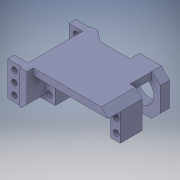
# Autodesk Inventor part: 000.502 - Стяжка
Saved by Autodesk Inventor 2019 (Build 230136000, 136)
## iProperties
Created: 2020-02-29
Part Number: 000.502 - Стяжка
Material: Пластик АБС
Document SubType Name: Modeling
Designer: Петров Иван
Density: 1.06 g/cm^3
Appearance: Грифельно-синий
Author: Петров Иван
Autodesk Inventor part; units mm, degrees
ref_plane "YZ Plane" through (0, 0, 0) normal (1, 0, 0) x (0, 1, 0)
ref_plane "XZ Plane" through (0, 0, 0) normal (0, 1, 0) x (-1, 0, 0)
ref_plane "XY Plane" through (0, 0, 0) normal (0, 0, 1) x (1, 0, 0)
sketch "Эскиз1" plane through (0, 0, 0) normal (0, 1, 0) x (-1, 0, 0)
  line L0 (-20.35, 18.35) -> (-20.35, 12.05)
  line L1 (-20.35, 12.05) -> (-26.35, 12.05)
  line L2 (-26.35, 9.45) -> (-26.35, 12.05)
  line L3 (-20.35, 9.45) -> (-26.35, 9.45)
  line L4 (-20.35, 9.45) -> (-20.35, -16.35)
  line L5 (-20.35, -16.35) -> (20.35, -16.35)
  line L6 (20.35, -16.35) -> (20.35, 9.45)
  line L7 (20.35, 9.45) -> (26.35, 9.45)
  line L8 (26.35, 9.45) -> (26.35, 12.05)
  line L9 (20.35, 12.05) -> (26.35, 12.05)
  line L10 (20.35, 12.05) -> (20.35, 18.35)
  line L11 (20.35, 18.35) -> (-10.35, 18.35)
  line L12 (-10.35, 18.35) -> (-20.35, 18.35)
  line L13 (26.35, 12.05) -> (27.35, 12.05)
  line L14 (26.35, 9.45) -> (26.35, 12.05)
  line L15 (26.35, 9.45) -> (27.35, 9.45)
  line L16 (27.35, 9.45) -> (27.35, 12.05)
  line L17 (-26.35, 12.05) -> (-27.35, 12.05)
  line L18 (-27.35, 9.45) -> (-27.35, 12.05)
  line L19 (-26.35, 9.45) -> (-27.35, 9.45)
  line L20 (-26.35, 9.45) -> (-26.35, 12.05)
  line L21 (-19.55, -17.15) -> (-18.4831, -17.15)
  line L22 (-18.4831, -17.15) -> (-17.3169, -17.15)
  line L23 (-17.3169, -17.15) -> (-15.85, -17.15)
  line L24 (-15.85, -17.15) -> (-15.85, -18.35)
  line L25 (15.85, -18.35) -> (-15.85, -18.35)
  line L26 (15.85, -17.15) -> (15.85, -18.35)
  line L27 (15.85, -17.15) -> (17.3169, -17.15)
  line L28 (17.3169, -17.15) -> (18.4831, -17.15)
  line L29 (18.4831, -17.15) -> (19.55, -17.15)
  line L30 (19.55, -17.15) -> (20.35, -16.35)
  line L31 (-20.35, -16.35) -> (20.35, -16.35)
  line L32 (-19.55, -17.15) -> (-20.35, -16.35)
  line L33 (15.85, -18.35) -> (18.35, -18.35)
  line L34 (-15.85, -18.35) -> (-18.35, -18.35)
  line L35 (18.35, -17.15) -> (18.35, -18.35)
  line L36 (18.35, -18.35) -> (19.55, -17.15)
  line L37 (-19.55, -17.15) -> (-19.65, -17.15)
  line L38 (-18.35, -18.35) -> (-19.55, -17.15)
  line L39 (-7.95, 26.65) -> (-12.75, 26.65)
  line L40 (-10.35, 18.35) -> (-20.35, 18.35)
  line L41 (-10.35, 26.65) -> (-10.35, 18.35)
  line L42 (-27.35, 9.45) -> (27.35, 9.45)
  line L43 (27.35, 9.45) -> (27.35, -19.4732)
  line L44 (27.35, -19.4732) -> (-27.35, -19.4732)
  line L45 (-27.35, -19.4732) -> (-27.35, 9.45)
  line L46 (20.35, 9.45) -> (-20.35, 9.45)
  line L47 (-20.35, 9.45) -> (-20.35, -18.35)
  line L48 (-20.35, -18.35) -> (20.35, -18.35)
  line L49 (20.35, -18.35) -> (20.35, 9.45)
  line L50 (-20.35, -16.35) -> (-27.35, -16.35)
  line L51 (-27.35, -16.35) -> (-27.35, -6.7017)
  line L52 (-27.35, -6.7017) -> (-20.35, -6.7017)
  line L53 (-20.35, -6.7017) -> (-20.35, -16.35)
  line L54 (27.35, -16.35) -> (27.35, -6.7017)
  line L55 (27.35, -6.7017) -> (20.35, -6.7017)
  line L56 (20.35, -6.7017) -> (20.35, -16.35)
  line L57 (27.35, 9.45) -> (20.35, 9.45)
  line L58 (20.35, 9.45) -> (20.35, -6.7017)
  line L59 (20.35, -6.7017) -> (27.35, -6.7017)
  line L60 (27.35, -6.7017) -> (27.35, 9.45)
  line L61 (-20.35, 9.45) -> (-27.35, 9.45)
  line L62 (-27.35, 9.45) -> (-27.35, -6.7017)
  line L63 (-27.35, -6.7017) -> (-20.35, -6.7017)
  line L64 (-20.35, -6.7017) -> (-20.35, 9.45)
  line L65 (27.35, -6.7017) -> (20.35, -6.7017)
  point P0 (0, 0)
  point P1 (0, 0)
  dimension "d0" = 0
  constraints: 132 end point, 12 equal length, 6 perpendicular, 5 horizontal, 4 point on line, 1 midpoint
  measures "d0" distance between parallel lines of L7 L42
extrude "Выдавливание1" add sketch "Эскиз1" along normal blind 20 contours L3 L4 L52 L45 L19 | L7 L15 L43 L55 L6
sketch "Эскиз2" plane through (0, 20, 0) normal (0, 1, 0) x (1, 0, 0)
  line L0 (-27.35, -9.45) -> (-20.35, -9.45) projected
  line L1 (27.35, -9.45) -> (27.35, 6.7017) projected
  line L2 (-27.35, -9.45) -> (27.35, -9.45)
  line L3 (27.35, -9.45) -> (27.35, 6.7017)
  line L4 (27.35, 6.7017) -> (-27.35, 6.7017)
  line L5 (-27.35, 6.7017) -> (-27.35, -9.45)
  point P0 (0, 0)
  constraints: 8 end point, 2 parallel, 1 horizontal, 1 perpendicular
extrude "Выдавливание2" add sketch "Эскиз2" along normal blind 5
sketch "Эскиз3" plane through (20.35, 0, 9.45) normal (0, 0, 1) x (1, 0, 0)
  line L0 (-47.7, 13.75) -> (-47.7, 10.5)
  line L1 (-47.7, 10.5) -> (-40.7, 10.5)
  line L2 (-40.7, 10.5) -> (-40.7, 20)
  line L3 (-40.7, 20) -> (-46.7, 20)
  arc A0 (-46.7, 20) -> (-47.7, 19) centre (-46.7, 19) ccw
  line L4 (-47.7, 19) -> (-47.7, 16.15)
  line L5 (-47.7, 16.15) -> (-46.634, 16.15)
  arc A1 (-46.634, 13.75) -> (-46.634, 16.15) centre (-44.85, 14.95) ccw
  line L6 (-46.634, 13.75) -> (-47.7, 13.75)
  line L7 (-47.7, 9.5) -> (-40.7, 9.5)
  line L8 (-47.7, 9.5) -> (-47.7, 6.25)
  line L9 (-47.7, 6.25) -> (-46.634, 6.25)
  arc A2 (-46.634, 3.85) -> (-46.634, 6.25) centre (-44.85, 5.05) ccw
  line L10 (-46.634, 3.85) -> (-47.7, 3.85)
  line L11 (-47.7, 3.85) -> (-47.7, 1)
  arc A3 (-47.7, 1) -> (-46.7, 0) centre (-46.7, 1) ccw
  line L12 (-46.7, 0) -> (-40.7, 0)
  line L13 (-40.7, 0) -> (-40.7, 9.5)
  line L14 (0, 9.5) -> (7, 9.5)
  line L15 (0, 0) -> (0, 9.5)
  line L16 (6, 0) -> (0, 0)
  arc A4 (6, 0) -> (7, 1) centre (6, 1) ccw
  line L17 (7, 3.85) -> (7, 1)
  line L18 (5.934, 3.85) -> (7, 3.85)
  arc A5 (5.934, 6.25) -> (5.934, 3.85) centre (4.15, 5.05) ccw
  line L19 (7, 6.25) -> (5.934, 6.25)
  line L20 (7, 9.5) -> (7, 6.25)
  line L21 (0, 10.5) -> (0, 20)
  line L22 (0, 10.5) -> (7, 10.5)
  line L23 (7, 13.75) -> (7, 10.5)
  line L24 (5.934, 13.75) -> (7, 13.75)
  arc A6 (5.934, 16.15) -> (5.934, 13.75) centre (4.15, 14.95) ccw
  line L25 (7, 16.15) -> (5.934, 16.15)
  line L26 (7, 19) -> (7, 16.15)
  arc A7 (7, 19) -> (6, 20) centre (6, 19) ccw
  line L27 (0, 20) -> (6, 20)
  line L28 (-40.7, 20) -> (-10, 20)
  line L29 (-10, 20) -> (0, 20)
  line L30 (-10, 0) -> (0, 0)
  line L31 (-40.7, 0) -> (-10, 0)
  circle A8 centre (-10, 10) radius 6.5
  circle A9 centre (-10, 10) radius 5.4
  circle A10 centre (-10, 10) radius 3.4957
  circle A11 centre (-10, 10) radius 3.4957
  circle A12 centre (-44.85, 14.95) radius 2.15
  circle A13 centre (-44.85, 5.05) radius 2.15
  arc A14 (5.934, 16.15) -> (5.934, 13.75) centre (4.15, 14.95) ccw
  circle A15 centre (4.15, 14.95) radius 2.15
  circle A16 centre (4.15, 5.05) radius 2.15
  line L32 (-47.7, 13.75) -> (-47.7, 10.5)
  line L33 (-47.7, 16.15) -> (-47.7, 13.75)
  line L34 (-47.7, 13.75) -> (-47.7, 6.25)
  line L35 (-47.7, 6.25) -> (-47.7, 3.85)
  line L36 (7, 16.15) -> (7, 13.75)
  line L37 (7, 6.25) -> (5.934, 6.25)
  line L38 (7, 6.25) -> (7, 3.85)
  line L39 (0, 20) -> (-40.7, 20) projected
  line L40 (-10, 20) -> (0, 20)
  point P0 (-20.35, 0)
  point P1 (-20.35, 0)
  constraints: 80 end point, 18 point on circle, 15 centre point, 4 coincident, 2 collinear, 2 concentric, 2 vertical, 1 perpendicular, 1 point on line, 6 other
extrude "Выдавливание3" cut sketch "Эскиз3" against normal through all contours A12 A1 | A2 A13 | A16 A5 | A6 A15
sketch "Эскиз4" plane through (0, 25, 0) normal (0, 1, 0) x (1, 0, 0)
  line L0 (20.35, -18.35) -> (20.35, -12.05)
  line L1 (20.35, -12.05) -> (26.35, -12.05)
  line L2 (26.35, -9.45) -> (26.35, -12.05)
  line L3 (20.35, -9.45) -> (26.35, -9.45)
  line L4 (20.35, -9.45) -> (20.35, 16.35)
  line L5 (-20.35, 16.35) -> (-20.35, -9.45)
  line L6 (-20.35, -9.45) -> (-26.35, -9.45)
  line L7 (-26.35, -9.45) -> (-26.35, -12.05)
  line L8 (-20.35, -12.05) -> (-26.35, -12.05)
  line L9 (-20.35, -12.05) -> (-20.35, -18.35)
  line L10 (-20.35, -18.35) -> (10.35, -18.35)
  line L11 (10.35, -18.35) -> (20.35, -18.35)
  line L12 (-26.35, -12.05) -> (-27.35, -12.05)
  line L13 (-26.35, -9.45) -> (-26.35, -12.05)
  line L14 (-26.35, -9.45) -> (-27.35, -9.45)
  line L15 (-27.35, -9.45) -> (-27.35, -12.05)
  line L16 (26.35, -12.05) -> (27.35, -12.05)
  line L17 (27.35, -9.45) -> (27.35, -12.05)
  line L18 (26.35, -9.45) -> (27.35, -9.45)
  line L19 (26.35, -9.45) -> (26.35, -12.05)
  line L20 (19.55, 17.15) -> (18.4831, 17.15)
  line L21 (18.4831, 17.15) -> (18.35, 17.15)
  line L22 (-15.85, 17.15) -> (-15.85, 18.35)
  line L23 (-15.85, 17.15) -> (-17.3169, 17.15)
  line L24 (-17.3169, 17.15) -> (-18.4831, 17.15)
  line L25 (-18.4831, 17.15) -> (-19.55, 17.15)
  line L26 (-19.55, 17.15) -> (-20.35, 16.35)
  line L27 (19.55, 17.15) -> (20.35, 16.35)
  line L28 (-15.85, 18.35) -> (-18.35, 18.35)
  line L29 (-18.35, 17.15) -> (-18.35, 18.35)
  line L30 (-18.35, 18.35) -> (-19.55, 17.15)
  line L31 (19.55, 17.15) -> (19.65, 17.15)
  line L32 (18.35, 18.35) -> (19.55, 17.15)
  line L33 (7.95, -26.65) -> (12.75, -26.65)
  line L34 (10.35, -18.35) -> (20.35, -18.35)
  line L35 (10.35, -26.65) -> (10.35, -18.35)
  line L36 (27.35, -9.45) -> (-27.35, -9.45)
  line L37 (-27.35, -9.45) -> (-27.35, 19.4732)
  line L38 (27.35, 19.4732) -> (27.35, -9.45)
  line L39 (-20.35, -9.45) -> (20.35, -9.45)
  line L40 (20.35, -9.45) -> (20.35, 18.35)
  line L41 (-20.35, 18.35) -> (-20.35, -9.45)
  line L42 (20.35, 16.35) -> (27.35, 16.35)
  line L43 (27.35, 16.35) -> (27.35, 6.7017)
  line L44 (27.35, 6.7017) -> (20.35, 6.7017)
  line L45 (20.35, 6.7017) -> (20.35, 16.35)
  line L46 (-27.35, 16.35) -> (-27.35, 6.7017)
  line L47 (-27.35, 6.7017) -> (-20.35, 6.7017)
  line L48 (-20.35, 6.7017) -> (-20.35, 16.35)
  line L49 (-27.35, -9.45) -> (-20.35, -9.45)
  line L50 (-20.35, -9.45) -> (-20.35, 6.7017)
  line L51 (-20.35, 6.7017) -> (-27.35, 6.7017)
  line L52 (-27.35, 6.7017) -> (-27.35, -9.45)
  line L53 (20.35, -9.45) -> (27.35, -9.45)
  line L54 (27.35, -9.45) -> (27.35, 6.7017)
  line L55 (27.35, 6.7017) -> (20.35, 6.7017)
  line L56 (20.35, 6.7017) -> (20.35, -9.45)
  line L57 (-27.35, 6.7017) -> (-20.35, 6.7017)
  line L58 (27.35, 6.7017) -> (-27.35, 6.7017) projected
  line L59 (10.35, 6.7017) -> (10.35, 29.7017)
  line L60 (10.35, 29.7017) -> (2.35, 29.7017)
  line L61 (2.35, 29.7017) -> (2.35, 6.7017)
  line L62 (2.35, 6.7017) -> (10.35, 6.7017)
  line L63 (10.35, 6.7017) -> (10.35, 29.7017)
  line L64 (10.35, 29.7017) -> (18.35, 29.7017)
  line L65 (18.35, 29.7017) -> (18.35, 6.7017)
  line L66 (18.35, 6.7017) -> (10.35, 6.7017)
  line L67 (10.35, 6.7017) -> (10.35, 29.7017)
  line L68 (-27.35, 19.4732) -> (-15.85, 19.4732)
  line L69 (18.35, 19.4732) -> (27.35, 19.4732)
  line L70 (20.35, 18.35) -> (18.35, 18.35)
  line L71 (-15.85, 18.35) -> (-20.35, 18.35)
  line L72 (20.35, 16.35) -> (18.35, 16.35)
  line L73 (-15.85, 16.35) -> (-20.35, 16.35)
  line L74 (20.35, 16.35) -> (18.35, 16.35)
  line L75 (-15.85, 16.35) -> (-20.35, 16.35)
  point P0 (0, 0)
  point P1 (0, 0)
  point P2 (0, 0)
  dimension "d7" = 0
  dimension "d8" = 23
  dimension "d9" = 8
  dimension "d10" = 8
  constraints: 150 end point, 17 parallel, 10 perpendicular, 10 point on line, 2 horizontal, 1 collinear, 1 midpoint, 4 other
  measures "d7" distance between parallel lines of L6 L36
  measures "d8" distance of L59.start L59.end
  measures "d9" distance of L62.end L61.end
  measures "d10" distance of L65.end L66.end
extrude "Выдавливание4" add sketch "Эскиз4" against normal blind 5 contours L58 L59 L64 L65 | L58 L61 L60 L59
sketch "Эскиз5" plane through (0, 20, 0) normal (0, -1, 0) x (1, 0, 0)
  line L0 (-3.65, -29.7017) -> (24.35, -29.7017)
  line L1 (24.35, -29.7017) -> (24.35, -22.7017)
  line L2 (24.35, -22.7017) -> (-3.65, -22.7017)
  line L3 (-3.65, -22.7017) -> (-3.65, -29.7017)
  line L4 (2.35, -29.7017) -> (18.35, -29.7017) projected
  line L5 (2.35, -6.7017) -> (2.35, -29.7017) projected
  point P0 (0, 0)
  dimension "d13" = 28
  dimension "d14" = 7
  dimension "d15" = 0
  dimension "d16" = 6
  constraints: 8 end point, 2 parallel, 1 horizontal, 1 perpendicular
  measures "d13" distance of L2.end L1.end
  measures "d14" distance of L1.end L0.end
  measures "d15" distance between parallel lines of L4 L0
  measures "d16" distance between parallel lines of L3 L5
extrude "Выдавливание5" add sketch "Эскиз5" along normal blind 25
sketch "Эскиз6" plane through (18.35, 25, -29.7017) normal (0, 0, -1) x (-1, 0, 0)
  line L0 (22, -30) -> (-6, -30) projected
  line L1 (8, -30) -> (8, -15)
  circle A0 centre (8, -15) radius 9.5
  point P0 (18.35, -25)
  dimension "d19" = 15
  dimension "d20" = 19
  constraints: 2 end point, 1 centre point, 1 coincident, 1 midpoint, 1 vertical
  measures "d19" distance of L1.start L1.end
  measures "d20" diameter of A0
extrude "Выдавливание6" cut sketch "Эскиз6" against normal blind 28
chamfer "Фаска1" distance 5 angle 45 2 edges at (18.35, 20, -26.2017) (2.35, 20, -26.2017)
chamfer "Фаска2" distance 1 angle 45 2 edges at (24.35, 20, -26.2017) (-3.65, 20, -26.2017)
chamfer "Фаска3" distance 6.25 angle 45 2 edges at (24.35, -5, -26.2017) (-3.65, -5, -26.2017)
sketch "Эскиз7" plane through (-27.35, 0, -6.7017) normal (-1, 0, 0) x (0, 0, 1)
  line L0 (-22.1483, 3.5419) -> (-22.1483, 30) projected
  line L1 (29.8517, 30) -> (29.8517, 3.5419) projected
  line L2 (3.8517, 25) -> (3.8517, 7.2)
  line L3 (16.1517, 7.2) -> (0, 7.2) projected
  line L4 (29.8517, 0) -> (29.8517, 25)
  line L5 (-22.1483, 30) -> (-22.1483, 0)
  line L6 (-22.1483, 0) -> (29.8517, 0)
  line L7 (-23, 25) -> (-16, 25) projected
  line L8 (-22.1483, 25) -> (29.8517, 25)
  point P0 (6.7017, 0)
  dimension "d40" = 0
  constraints: 10 end point, 3 point on line, 2 perpendicular, 1 midpoint, 1 parallel
  measures "d40" distance from line of point (6.702, 0) L6
extrude "Выдавливание7" add sketch "Эскиз7" along normal blind 5
chamfer "Фаска5" distance 15.5 angle 45 1 edges at (2.35, 22.5, -6.7017)
sketch "Эскиз8" plane through (-32.35, 0, -6.7017) normal (-1, 0, 0) x (0, 0, 1)
  line L0 (-22.1483, 3.5419) -> (-22.1483, 30)
  line L1 (29.8517, 30) -> (29.8517, 3.5419)
  line L2 (29.8517, 0) -> (29.8517, 25)
  line L3 (-22.1483, 30) -> (-22.1483, 0)
  line L4 (-22.1483, 0) -> (29.8517, 0)
  line L5 (-23, 25) -> (-16, 25)
  line L6 (-22.1483, 25) -> (29.8517, 25)
  line L7 (3.8517, 25) -> (3.8517, 0)
  line L8 (16.1517, 0) -> (0, 0) projected
  line L9 (3.8517, 12.5) -> (-16.1483, 12.5)
  line L10 (-23, 25) -> (-16, 25) projected
  line L11 (-21.1483, 12.5) -> (-21.1483, 25)
  line L12 (-21.1483, 25) -> (-16.1483, 25)
  line L13 (-16.1483, 25) -> (-16.1483, 12.5)
  line L14 (-21.1483, 12.5) -> (-21.1483, 0)
  line L15 (-22.1483, 0) -> (0, 0) projected
  line L16 (-16.1483, 12.5) -> (-16.1483, 0)
  point P0 (6.7017, 0)
  point P1 (6.7017, 0)
  dimension "d41" = 0
  dimension "d42" = 20
  dimension "d43" = 5
  constraints: 28 end point, 6 point on line, 4 perpendicular, 2 midpoint, 2 parallel, 2 vertical, 1 horizontal
  measures "d41" distance from line of point (6.702, 0) L4
  measures "d42" distance of L9.start L9.end
  measures "d43" distance of L11.end L12.end
extrude "Выдавливание8" add sketch "Эскиз8" along normal blind 10 contours L5 L13 L16 L4 L14 L11
sketch "Эскиз9" plane through (-32.35, 0, -27.85) normal (0, 0, -1) x (-1, 0, 0)
  line L0 (10, 0) -> (10, 25) projected
  line L1 (10, 12.5) -> (5, 12.5)
  circle A0 centre (5, 12.5) radius 2
  point P0 (-32.35, 0)
  dimension "d46" = 5
  dimension "d47" = 4
  constraints: 2 end point, 1 centre point, 1 coincident, 1 horizontal, 1 midpoint
  measures "d46" distance of L1.start L1.end
  measures "d47" diameter of A0
extrude "Выдавливание9" cut sketch "Эскиз9" against normal blind 8
pattern_linear "Прямоуг.массив1" count 3 spacing 8 along (0, -1, 0) of "Выдавливание9" first direction both ways yes
sketch "Эскиз10" plane through (-32.35, 0, -6.7017) normal (-1, 0, 0) x (0, 0, 1)
  line L0 (-22.1483, 3.5419) -> (-22.1483, 30)
  line L1 (29.8517, 30) -> (29.8517, 3.5419)
  line L2 (3.8517, 25) -> (3.8517, 7.2)
  line L3 (16.1517, 7.2) -> (0, 7.2)
  line L4 (29.8517, 0) -> (29.8517, 25)
  line L5 (-22.1483, 30) -> (-22.1483, 0)
  line L6 (-22.1483, 0) -> (29.8517, 0)
  line L7 (-23, 25) -> (-16, 25)
  line L8 (-22.1483, 25) -> (29.8517, 25)
  point P0 (6.7017, 0)
  point P1 (6.7017, 0)
  dimension "d53" = 0
  constraints: 18 end point, 3 point on line, 2 perpendicular, 1 midpoint, 1 parallel
  measures "d53" distance from line of point (6.702, 0) L6
ref_plane "РабПлоскость1" through (-32.35, 25, -2.85) normal (0, 0, -1) x (0, -1, 0)
mirror "Зеркальное отражение1" about plane through (-32.35, 25, -2.85) normal (0, 0, -1) of "Выдавливание9", "Прямоуг.массив1", "Выдавливание8"
chamfer "Фаска6" distance 4 angle 45 2 edges at (-27.35, 0, -17.7758) (-27.35, 0, 16.3)
chamfer "Фаска7" distance 7.25 angle 45 1 edges at (-13.15, 22.5, -6.7017)
chamfer "Фаска8" distance 13.25 angle 45 1 edges at (-8.0235, 22.5, -11.8282)
sketch "Эскиз12" plane through (0, 25, 0) normal (0, 1, 0) x (1, 0, 0)
  line L0 (2.35, 29.7017) -> (2.35, 22.7017) projected
  line L1 (-27.35, 6.7017) -> (-27.35, 28.85) projected
  line L2 (2.35, 22.7017) -> (-27.35, 22.7017)
  line L3 (-27.35, 22.7017) -> (-27.35, 6.7017)
  line L4 (-27.35, 6.7017) -> (2.35, 6.7017)
  line L5 (2.35, 6.7017) -> (2.35, 22.7017)
  point P0 (0, 0)
  constraints: 8 end point, 2 parallel, 1 horizontal, 1 perpendicular
extrude "Выдавливание11" add sketch "Эскиз12" against normal up to surface (5 mm away)
chamfer "Фаска10" distance 5 angle 45 1 edges at (27.35, 25, 1.3742)
chamfer "Фаска11" distance 6 distance2 7.75 1 edges at (-27.35, 22.5, -22.7017) measured on face at (-27.35, 22.5, -23.2017)
chamfer "Фаска12" distance 2 angle 45 1 edges at (-27.35, 14.5, -28.85)
sketch "Эскиз13" plane through (20.35, 0, 9.45) normal (0, 0, 1) x (1, 0, 0)
  line L0 (2, 25) -> (7, 20) projected
  line L1 (-49.7, 20) -> (-47.7, 20) projected
  line L2 (-47.8916, 20) -> (-47.8916, 25) projected
  line L3 (-47.7, 20) -> (-47.7, 25)
  line L4 (-47.7, 25) -> (2, 25) projected
  line L5 (-47.7, 25) -> (2, 25)
  line L6 (2, 25) -> (7, 20)
  line L7 (7, 20) -> (-47.7, 20)
  line L8 (-2, 20) -> (-23, 20) projected
  point P0 (-20.35, 0)
  point P1 (-40.7, 20)
  point P2 (-39.95, 20)
  constraints: 8 end point, 3 collinear, 1 parallel
extrude "Выдавливание12" add sketch "Эскиз13" along normal blind 8.9
